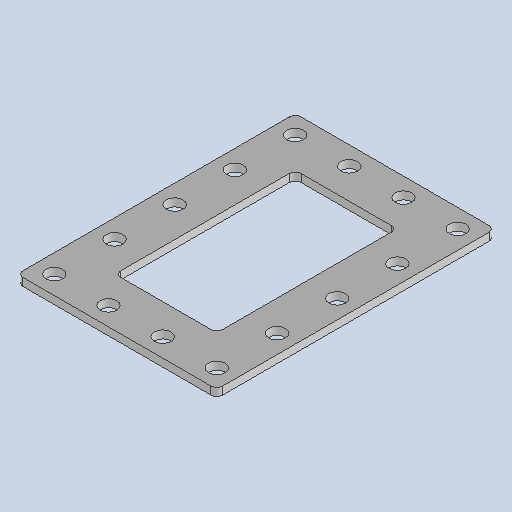
# Autodesk Inventor part: PRS 9606 charging flange round_D1200 940
Saved by Autodesk Inventor 2026.2 (Build 302298000, 298)
## iProperties
Created: 2025-02-13
Part Number: PRS 9606 charging flange round_D1200 940
Material: Steel
Document SubType Name: Sheet Metal
Designer: admin
Mass: 2237.08 g
Surface Area: 894.773 cm^2
Volume: 284.978 cm^3
Density: 7.85 g/cm^3
Flat Pattern Width: 28.4 cm
Flat Pattern Length: 20.4 cm
Flat Pattern Area: 579.36 cm^2
Sheet Metal Rule: AISI304 4mm Die 32
Sheet Metal Width: 284,000 mm
Sheet Metal Length: 204,000 mm
Sheet Metal Area: 57936,000 mm^2
Appearance: Default
Author: pokla
Autodesk Inventor part; units mm, degrees
ref_plane "YZ Plane" through (0, 0, 0) normal (1, 0, 0) x (0, 1, 0)
ref_plane "XZ Plane" through (0, 0, 0) normal (0, 1, 0) x (-1, 0, 0)
ref_plane "XY Plane" through (0, 0, 0) normal (0, 0, 1) x (1, 0, 0)
sketch "Sketch2" plane through (0, 0, 0) normal (0, 0, 1) x (1, 0, 0)
  line L0 (-52, -92) -> (52, -92)
  line L1 (52, -92) -> (52, 92)
  line L2 (52, 92) -> (-52, 92)
  line L3 (-52, 92) -> (-52, -92)
  line L4 (-52, -92) -> (52, 92) construction
  line L5 (52, -92) -> (-52, 92) construction
  line L6 (-102, -142) -> (102, -142)
  line L7 (102, -142) -> (102, 142)
  line L8 (102, 142) -> (-102, 142)
  line L9 (-102, 142) -> (-102, -142)
  point P0 (0, 0)
  dimension "d29" = 104
  dimension "d30" = 184
  dimension "d31" = 50
  measures "d29" distance of L2.end L1.end
  measures "d30" distance of L1.end L0.end
  measures "d31" distance between parallel lines of L3 L9
extrude "Plate2" add sketch "Sketch2" along normal blind 8
sketch "Sketch5" plane through (0, 0, 8) normal (0, 0, 1) x (1, 0, 0)
  line L0 (52, 92) -> (52, -92) construction
  line L1 (52, -92) -> (-52, -92) construction
  line L2 (-52, -92) -> (-52, 92) construction
  line L3 (-52, 92) -> (52, 92) construction
  line L4 (102, -142) -> (-102, -142) construction
  line L5 (102, 142) -> (102, -142) construction
  line L6 (-102, 142) -> (102, 142) construction
  line L7 (-102, -142) -> (-102, 142) construction
  line L8 (-83, 123) -> (83, 123) construction
  line L9 (83, 123) -> (83, -123) construction
  line L10 (83, -123) -> (-83, -123) construction
  line L11 (-83, -123) -> (-83, 123) construction
  line L12 (-52, 0) -> (52, 0) construction
  line L13 (0, 92) -> (0, -92)
  point P0 (0, 0)
  point P1 (0, -123)
  point P2 (-83, 61.5)
  point P3 (-83, 0)
  point P4 (-83, -61.5)
  point P5 (-27.6667, -123)
  point P6 (27.6667, -123)
  point P7 (83, -61.5)
  point P8 (83, 0)
  point P9 (83, 61.5)
  point P10 (27.6667, 123)
  point P11 (-27.6667, 123)
  dimension "d34" = 19
  dimension "d49" = 61.5
  dimension "d50" = 61.5
  dimension "d51" = 55.3333
  dimension "d52" = 55.3333
  dimension "d53" = 55.3333
  constraints: 12 end point, 8 point on line, 7 midpoint, 4 coincident, 3 symmetric about line, 2 vertical alignment, 1 horizontal alignment, 3 other
  measures "d34" distance between parallel lines of L4 L10
  measures "d49" distance of point (-83, 61.5) point (-83, 123)
  measures "d50" distance of point (-83, 0) point (-83, 61.5)
  measures "d51" distance of point (-27.667, 123) point (-83, 123)
  measures "d52" distance of point (27.667, 123) point (-27.667, 123)
  measures "d53" distance of point (83, 123) point (27.667, 123)
fillet "Corner Round1" radius 6 8 edges at (-102, -142, 4) (-102, 142, 4) (102, 142, 4) (102, -142, 4) (52, -92, 4) (-52, -92, 4) (-52, 92, 4) (52, 92, 4)
hole "Hole1" at (-83, 123, 8) at (-83, 61.5, 8) at (-83, 0, 8) at (-83, -61.5, 8) at (-83, -123, 8) at (-27.6667, -123, 8) at (27.6667, -123, 8) at (83, -123, 8) at (83, -61.5, 8) at (83, 0, 8) at (83, 61.5, 8) at (83, 123, 8) at (27.6667, 123, 8) at (-27.6667, 123, 8) direction (0, 0, -1) diameter 17 end through all
equation "\"d49\" = d50"
equation "\"d51\" = d53"
equation "\"d52\" = d53"
equation "\"d29\" = ChargingHatch_hight - 2 * Thickness"
equation "\"d30\" = ChargingHatch_width - 2 * Thickness"
equation "\"d59\" = Thickness"
equation "\"d14\" = Thickness"
equation "\"BendReliefWidth\" = Thickness"
equation "\"BendReliefDepth\" = 0.5 * Thickness"
equation "\"CornerReliefSize\" = 4 * Thickness"
equation "\"MinimumRemnant\" = 2 * Thickness"
equation "\"TransitionRadius\" = BendRadius"
equation "\"JacobiRadiusSize\" = BendRadius"
equation "\"GapSize\" = Thickness"
equation "\"ChargingHatch_hight\" = 120"
equation "\"Thickness\" = 8"
equation "\"ChargingHatch_width\" = 200"
equation "\"BendRadius\" = 6"
body "Solid3"
